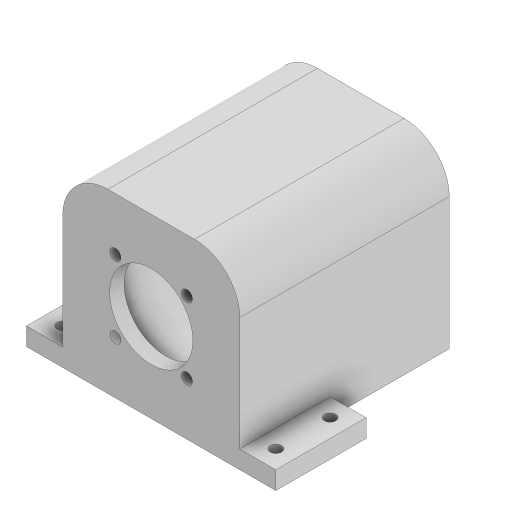
# Autodesk Inventor part: StepperMotorHolder
Saved by Autodesk Inventor 2023 (Build 270158000, 158)
## iProperties
Created: 2022-10-20
Part Number: StepperMotorHolder
Material: Generic
Document SubType Name: Modeling
Designer: MVeszpremi
Density: 1 g/cm^3
Appearance: Default
Author: MVeszpremi
Autodesk Inventor part; units mm, degrees
ref_plane "YZ Plane" through (0, 0, 0) normal (1, 0, 0) x (0, 1, 0)
ref_plane "XZ Plane" through (0, 0, 0) normal (0, 1, 0) x (-1, 0, 0)
ref_plane "XY Plane" through (0, 0, 0) normal (0, 0, 1) x (1, 0, 0)
sketch "Sketch1" plane through (0, 0, 0) normal (0, 0, 1) x (1, 0, 0)
  line L0 (-21.5, -21.5) -> (21.5, -21.5)
  line L1 (21.5, -21.5) -> (21.5, 21.5)
  line L2 (21.5, 21.5) -> (-21.5, 21.5)
  line L3 (-21.5, 21.5) -> (-21.5, -21.5)
  line L4 (-21.5, -21.5) -> (21.5, 21.5) construction
  line L5 (21.5, -21.5) -> (-21.5, 21.5) construction
  circle A0 centre (0, 0) radius 18.5
  circle A1 centre (0, 0) radius 11.5
  circle A2 centre (0, 0) radius 14
  circle A3 centre (-9.8995, 9.8995) radius 1.5
  circle A4 centre (-9.8995, -9.8995) radius 1.5
  circle A5 centre (9.8995, -9.8995) radius 1.5
  circle A6 centre (9.8995, 9.8995) radius 1.5
  line L6 (0, 0) -> (0, 21.5)
  line L7 (-24.5, 24.5) -> (24.5, 24.5)
  line L8 (24.5, 24.5) -> (24.5, -24.5)
  line L9 (24.5, -24.5) -> (-24.5, -24.5)
  line L10 (-24.5, -24.5) -> (-24.5, 24.5)
  line L11 (-24.5, 24.5) -> (24.5, -24.5) construction
  line L12 (24.5, 24.5) -> (-24.5, -24.5) construction
  dimension "d4" = 28
  dimension "d0" = 43
  dimension "d1" = 43
  dimension "d2" = 37
  dimension "d3" = 23
  dimension "d5" = 3
  dimension "d8" = 360
  dimension "d10" = 3
  dimension "d11" = 3
  constraints: 26 end point, 6 centre point, 5 midpoint, 4 parallel, 3 coincident, 2 horizontal, 2 perpendicular, 1 point on line, 12 other
  measures "d0" distance of L1.end L2.end
  measures "d1" distance of L2.end L0.start
  measures "d2" diameter of A0
  measures "d3" diameter of A1
  measures "d5" diameter of A3
  measures "d10" distance between parallel lines of L10 L3
  measures "d11" distance between parallel lines of L9 L0
extrude "Extrusion1" add sketch "Sketch1" along normal blind 5 and the other way blind 30 contours L7 L8 L9 L10
extrude "Extrusion2" add sketch "Sketch1" along normal blind 24 contours L3 L2 L1 L0
sketch "Sketch2" plane through (0, 0, 24) normal (0, 0, 1) x (1, 0, 0)
  circle A0 centre (0, 0) radius 11.5 projected
  circle A1 centre (0, 0) radius 14 projected
  circle A2 centre (9.8995, 9.8995) radius 1.5 projected
  circle A3 centre (9.8995, -9.8995) radius 1.5 projected
  circle A4 centre (-9.8995, -9.8995) radius 1.5 projected
  circle A5 centre (-9.8995, 9.8995) radius 1.5 projected
  circle A6 centre (0, 0) radius 18.5 projected
  line L0 (-21.5, 21.5) -> (-21.5, -21.5) projected
  line L1 (-21.5, -21.5) -> (21.5, -21.5) projected
  line L2 (21.5, -21.5) -> (21.5, 21.5) projected
  line L3 (21.5, 21.5) -> (-21.5, 21.5) projected
  circle A7 centre (0, 0) radius 18.5 projected
  line L4 (24.5, -24.5) -> (-24.5, -24.5) projected
  line L5 (24.5, 24.5) -> (24.5, -24.5) projected
  line L6 (-24.5, 24.5) -> (24.5, 24.5) projected
  line L7 (-24.5, -24.5) -> (-24.5, 24.5) projected
  line L8 (21.5, -21.5) -> (21.5, 21.5) projected
  line L9 (-21.5, -21.5) -> (21.5, -21.5) projected
  line L10 (-21.5, 21.5) -> (-21.5, -21.5) projected
  line L11 (21.5, 21.5) -> (-21.5, 21.5) projected
extrude "Extrusion3" add sketch "Sketch2" along normal blind 4 contours A1 A3 A4 A5 A2 | A6 | L3 L2 L1 L0
sketch "Sketch8" plane through (0, 0, 28) normal (0, 0, 1) x (1, 0, 0)
  line L0 (-24.5, -24.5) -> (24.5, -24.5) projected
  line L1 (24.5, -24.5) -> (24.5, 24.5) projected
  line L2 (24.5, 24.5) -> (-24.5, 24.5) projected
  line L3 (-24.5, 24.5) -> (-24.5, -24.5) projected
  line L4 (21.5, 21.5) -> (21.5, -21.5) projected
  line L5 (21.5, -21.5) -> (-21.5, -21.5) projected
  line L6 (-21.5, -21.5) -> (-21.5, 21.5) projected
  line L7 (-21.5, 21.5) -> (21.5, 21.5) projected
  line L8 (-21.5, 21.5) -> (-21.5, -21.5) projected
  line L9 (-21.5, -21.5) -> (21.5, -21.5) projected
  line L10 (21.5, -21.5) -> (21.5, 21.5) projected
  line L11 (21.5, 21.5) -> (-21.5, 21.5) projected
  circle A0 centre (-9.8995, 9.8995) radius 1.5 projected
  circle A1 centre (-9.8995, -9.8995) radius 1.5 projected
  circle A2 centre (9.8995, -9.8995) radius 1.5 projected
  circle A3 centre (0, 0) radius 11.5 projected
  circle A4 centre (9.8995, 9.8995) radius 1.5 projected
extrude "Extrusion8" add sketch "Sketch8" against normal up to surface (23 mm away) contours L3 L2 L1 L0
sketch "Sketch9" plane through (-24.5, -24.5, -30) normal (0, -1, 0) x (1, 0, 0)
  line L0 (49, 0) -> (49, 58) projected
  line L1 (49, 58) -> (59, 58)
  line L2 (59, 58) -> (59, 33)
  line L3 (59, 33) -> (49, 33)
  line L4 (49, 33) -> (49, 58)
  line L5 (0, 58) -> (0, 0) projected
  line L6 (0, 58) -> (-10, 58)
  line L7 (-10, 58) -> (-10, 33)
  line L8 (-10, 33) -> (0, 33)
  line L9 (0, 33) -> (0, 58)
  line L10 (0, 58) -> (49, 58) projected
  circle A0 centre (54, 38) radius 1.55
  circle A1 centre (54, 53) radius 1.55
  circle A2 centre (-5, 38) radius 1.55
  circle A3 centre (-5, 53) radius 1.55
  point P0 (24.5, 30)
  point P1 (0, 33)
  point P2 (49, 33)
  dimension "d72" = 0
  dimension "d73" = 25
  dimension "d74" = 25
  dimension "d75" = 10
  dimension "d76" = 10
  dimension "d77" = 15
  dimension "d78" = 15
  dimension "d79" = 5
  dimension "d80" = 5
  dimension "d81" = 3.1
  dimension "d82" = 3.1
  dimension "d83" = 3.1
  dimension "d84" = 3.1
  constraints: 16 end point, 4 centre point, 4 parallel, 3 point on line, 2 horizontal, 2 perpendicular, 2 vertical alignment
  measures "d72" distance between parallel lines of L1 L10
  measures "d73" distance of L1.end L2.end
  measures "d74" distance of L6.end L7.end
  measures "d75" distance of L7.end L8.end
  measures "d76" distance of L2.end L3.end
  measures "d77" distance of A1.centre A0.centre
  measures "d78" distance of A2.centre A3.centre
  measures "d79" horizontal distance of L7.end A2.centre
  measures "d80" distance from line of L3 A0.centre
  measures "d81" diameter of A0
  measures "d82" diameter of A1
  measures "d83" diameter of A2
  measures "d84" diameter of A3
extrude "Extrusion9" add sketch "Sketch9" against normal blind 5
chamfer "Chamfer3" distance 3.5 angle 45 2 edges at (21.5, 21.5, -15) (-21.5, 21.5, -15)
fillet "Fillet10" radius 12.5 2 edges at (-24.5, 24.5, -1) (24.5, 24.5, -1)
body "Solid1"
